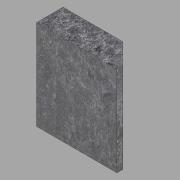
# Autodesk Inventor part: 3-80
Saved by Autodesk Inventor 2022.2 (Build 262287000, 287)
## iProperties
Created: 2021-12-23
Part Number: 3-80
Material: Granite, Cut, Polished
Document SubType Name: Modeling
Designer: awelt
Density: 2.7 g/cm^3
Appearance: Kasota SN sapphire
Mass: 4654.63 g
Surface Area: 1019.23 cm^2
Volume: 1723.94 cm^3
Author: awelt
Autodesk Inventor part; units mm, degrees
ref_plane "YZ Plane" through (0, 0, 0) normal (1, 0, 0) x (0, 1, 0)
ref_plane "XZ Plane" through (0, 0, 0) normal (0, 1, 0) x (-1, 0, 0)
ref_plane "XY Plane" through (0, 0, 0) normal (0, 0, 1) x (1, 0, 0)
sketch "Sketch1" plane through (0, 0, 0) normal (1, 0, 0) x (0, 1, 0)
  line L0 (0, 0) -> (57.15, 0)
  line L1 (57.15, 0) -> (57.15, 193.675)
  line L2 (57.15, 193.675) -> (0, 193.675)
  line L3 (0, 193.675) -> (0, 0)
  dimension "d0" = 57.15
  dimension "d1" = 193.675
  constraints: 8 end point, 2 parallel, 1 horizontal, 1 perpendicular
  measures "d0" distance of L2.end L1.end
  measures "d1" distance of L1.end L0.end
extrude "Extrusion1" add sketch "Sketch1" along normal blind 173.0375
sketch "Sketch3" plane through (0, 0, 0) normal (0, 0, -1) x (-1, 0, 0)
  line L0 (-173.0375, 57.15) -> (-173.0375, 0) projected
  line L1 (-173.0375, 44.45) -> (-128.5875, 0)
  line L2 (-173.0375, 44.45) -> (-110.1757, 44.45) construction
  line L3 (-128.5875, 0) -> (-173.0375, 0)
  line L4 (-173.0375, 0) -> (-173.0375, 44.45)
  point P0 (0, 0)
  dimension "d9" = 45
  dimension "d10" = 12.7
  dimension "d11" = 44.45
  constraints: 8 end point, 2 horizontal, 1 equal length, 1 perpendicular, 1 point on line
  measures "d9" angle of L1 L2
  measures "d10" distance of L1.start L0.start
  measures "d11" distance of L1.start L3.end
extrude "Extrusion3" cut sketch "Sketch3" against normal up to surface (193.675 mm away)
body "Solid1"
